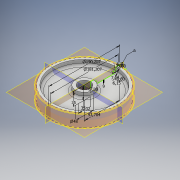
# Autodesk Inventor part: Колесо быстроходное
Saved by Autodesk Inventor 2018 (Build 220112000, 112)
## iProperties
Created: 2018-03-25
Part Number: Колесо быстроходное
Material: Типовые
Document SubType Name: Modeling
Designer: kriku
Density: 1 g/cm^3
Appearance: По умолчанию
Author: kriku
Autodesk Inventor part; units mm, degrees
sketch "Эскиз1" plane through (0, 0, 0) normal (1, 0, 0) x (0, 1, 0)
  line L0 (2.1047, 17.0457) -> (2.1047, -17.9543)
  line L1 (18.1047, 17.0457) -> (18.1047, -17.9543)
  line L2 (92.7082, -17.9543) -> (92.7082, 17.0457)
  line L3 (95.8082, 17.0457) -> (95.8082, -17.9543)
  line L4 (97.2082, 15.8457) -> (97.2082, -16.7543)
  line L5 (92.7082, 17.0457) -> (86.5582, 17.0457)
  line L6 (86.5582, 17.0457) -> (86.5582, 4.0457)
  line L7 (79.6537, 4.0457) -> (33.0093, 4.0457)
  line L8 (26.1047, 4.0457) -> (26.1047, 17.0457)
  line L9 (26.1047, 17.0457) -> (18.1047, 17.0457)
  line L10 (92.7082, -17.9543) -> (86.5582, -17.9543)
  line L11 (86.5582, -17.9543) -> (86.5582, -4.9543)
  line L12 (79.6537, -4.9543) -> (33.0093, -4.9543)
  line L13 (26.1047, -4.9543) -> (26.1047, -17.9543)
  line L14 (26.1047, -17.9543) -> (18.1047, -17.9543)
  line L15 (114.0861, -0.4543) -> (-18.3135, -0.4543)
  line L16 (96.0082, 17.0457) -> (92.7082, 17.0457)
  line L17 (96.0082, -17.9543) -> (92.7082, -17.9543)
  line L18 (26.1047, -17.9543) -> (27.054, -10.2231)
  line L19 (86.5582, -17.9543) -> (85.609, -10.2231)
  line L20 (86.5582, 17.0457) -> (85.609, 9.3145)
  line L21 (26.1047, 17.0457) -> (27.054, 9.3145)
  arc A0 (85.609, -10.2231) -> (79.6537, -4.9543) centre (79.6537, -10.9543) ccw
  arc A1 (33.0093, -4.9543) -> (27.054, -10.2231) centre (33.0093, -10.9543) ccw
  arc A2 (27.054, 9.3145) -> (33.0093, 4.0457) centre (33.0093, 10.0457) ccw
  arc A3 (79.6537, 4.0457) -> (85.609, 9.3145) centre (79.6537, 10.0457) ccw
  line L22 (97.2082, 15.8457) -> (96.0082, 17.0457)
  line L23 (97.2082, -16.7543) -> (96.0082, -17.9543)
  point P0 (0, 0)
  dimension "d0" = 35
  dimension "d1" = 32
  dimension "d3" = 35
  dimension "d4" = 9
  dimension "d5" = 181.207
  dimension "d6" = 93.7035
  dimension "d7" = 190.207
  dimension "d9" = 6.15
  dimension "d10" = 48
  dimension "d11" = 7
  dimension "d12" = 7
  dimension "d13" = 7
  dimension "d14" = 6
  dimension "d15" = 6
  dimension "d16" = 135
  dimension "d17" = 1.2
  dimension "d18" = 135
  dimension "d19" = 1.2
  constraints: 48 end point, 10 point on line, 8 point on circle, 8 tangent, 7 perpendicular, 4 centre point, 4 parallel, 4 vertical, 2 equal radius, 2 horizontal, 2 symmetric about line, 2 other
  measures "d0" distance of L0.start L0.end
  measures "d1" diameter of L1 L0
  measures "d3" distance of L1.start L1.end
  measures "d4" distance between parallel lines of L12 L7
  measures "d5" diameter of L2 L0
  measures "d6" distance between parallel lines of L0 L3
  measures "d7" diameter of L4 L0
  measures "d9" distance from line of L10.end L2
  measures "d10" diameter of L13 L0
  measures "d11" angle of L11 L19
  measures "d12" angle of L20 L6
  measures "d13" angle of L13 L18
  measures "d14" radius of A0
  measures "d15" radius of A1
  measures "d16" angle of L4 L22
  measures "d17" horizontal distance of L16.start L4.start
  measures "d18" angle of L4 L23
  measures "d19" horizontal distance of L4.end L17.start
revolve "Вращение1" add sketch "Эскиз1" angle 360 about axis through (0, 2.1047, 17.0457) along (0, 0, -1) contours L9 L21 A2 L7 A3 L20 L5 L2 L15 L1 | L15 L2 L10 L19 A0 L12 A1 L18 L14 L1
surface revolve "ВращПврх1" sketch "Эскиз1" angle 360 about axis through (0, 2.1047, 17.0457) along (0, 0, -1) shown yes curves L16 L22 L4 L23 L17
body "SRF1"
